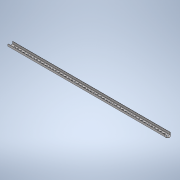
# Autodesk Inventor part: HalfBeam
Saved by Autodesk Inventor 2022 (Build 260153000, 153)
## iProperties
Created: 2022-04-08
Part Number: HalfBeam
Material: Steel, Mild, Welded
Document SubType Name: Sheet Metal
Designer: Patrick
Density: 7.85 g/cm^3
Sheet Metal Rule: Default_mm
Appearance: Weld - Steel Mild
Flat Pattern Width: 5.47858 cm
Flat Pattern Length: 100 cm
Flat Pattern Area: 547.858 cm^2
Sheet Metal Width: 54,786 mm
Sheet Metal Length: 1000,000 mm
Sheet Metal Area: 54785,840 mm^2
Mass: 576.831 g
Surface Area: 1040.14 cm^2
Volume: 73.4817 cm^3
Author: Patrick
Autodesk Inventor part; units mm, degrees
ref_plane "YZ Plane" through (0, 0, 0) normal (1, 0, 0) x (0, 1, 0)
ref_plane "XZ Plane" through (0, 0, 0) normal (0, 1, 0) x (-1, 0, 0)
ref_plane "XY Plane" through (0, 0, 0) normal (0, 0, 1) x (1, 0, 0)
sketch "Sketch1" plane through (0, 0, 0) normal (0, 1, 0) x (-1, 0, 0)
  line L0 (0, 0) -> (1000, 0)
  line L1 (1000, 0) -> (1000, -30)
  line L2 (1000, -30) -> (0, -30)
  line L3 (0, -30) -> (0, 0)
  dimension "d0" = 1000
  dimension "d1" = 30
  measures "d0" distance of L1.end L2.end
  measures "d1" distance of L0.end L1.end
extrude "Plate1" add sketch "Sketch1" along normal blind 1.5
sketch "Sketch2" plane through (0, 0, -1.5) normal (0, 0, 1) x (1, 0, 0)
  line L0 (-1000, 0) -> (0, 0)
  line L1 (0, 0) -> (0, 15)
  line L2 (0, 15) -> (-1000, 15)
  line L3 (-1000, 15) -> (-1000, 0)
  constraints: 6 end point, 1 horizontal, 1 perpendicular, 1 vertical
edge flange "Flange1" height 15 angle 90 thickness 1.5 bend radius 1.5 thickness toward (0, 0, 1) relief tear relief width 1.5 relief depth 0.75 corner gap 1.5 corner form 0 edges at (-500, 1.5, 0) (-500, 1.5, -30) wall of the first edge with corners at (-1000, 0, -1.5) (0, 0, -1.5) (0, 15, -1.5) (-1000, 15, -1.5)
bend "Bend1"
corner "Corner1"
sketch "Sketch3" plane through (0, 1.5, 0) normal (0, 1, 0) x (1, 0, 0)
  circle A0 centre (-15, 15) radius 6.1
  line L0 (0, 27) -> (0, 3) projected
  line L1 (-1000, 0) -> (0, 0) projected
  dimension "d13" = 15
  dimension "d14" = 15
  dimension "d22" = 12.2
  constraints: 1 centre point
  measures "d13" distance from line of L0 A0.centre
  measures "d14" distance from line of L1 A0.centre
  measures "d22" diameter of A0
extrude "Extrusion1" cut sketch "Sketch3" against normal through all
pattern_linear "Rectangular Pattern1" count 49 spacing 20 along (-1, 0, 0) of "Extrusion1"
sketch "Sketch4" plane through (0, 0, 0) normal (0, -1, 0) x (1, 0, 0)
  line L0 (0, -30) -> (-1000, -30) projected
  line L1 (-1000, 0) -> (0, 0) projected
  arc A0 (-14.888, -30) -> (-14.888, 0) centre (-14.888, -15) ccw
  line L2 (-14.888, 0) -> (0, 0)
  line L3 (0, -30) -> (0, 0)
  line L4 (0, -30) -> (-15.1128, -30)
  point P0 (0, -16.8293)
  point P1 (0, -13.1707)
  constraints: 6 end point, 3 point on line, 2 point on circle, 1 centre point, 1 collinear, 1 perpendicular, 1 tangent
extrude "Extrusion2" cut sketch "Sketch4" against normal through all contours A0 L1 L3 | L0 A0 L3
equation "\"d2\" = Thickness"
equation "\"d3\" = BendReliefWidth"
equation "\"d4\" = BendReliefDepth"
equation "\"d5\" = MinimumRemnant"
equation "\"d6\" = TransitionRadius"
equation "\"d9\" = BendRadius"
equation "\"d10\" = CornerReliefSize"
equation "\"d11\" = GapSize"
equation "\"d12\" = JacobiRadiusSize"
equation "\"BendRadius\" = Thickness"
equation "\"BendReliefWidth\" = Thickness"
equation "\"BendReliefDepth\" = 0.5 * Thickness"
equation "\"CornerReliefSize\" = 4 * Thickness"
equation "\"MinimumRemnant\" = 2 * Thickness"
equation "\"TransitionRadius\" = BendRadius"
equation "\"JacobiRadiusSize\" = BendRadius"
equation "\"GapSize\" = Thickness"
equation "\"Thickness\" = 1.5"
body "Solid1"
